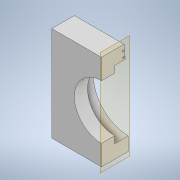
# Autodesk Inventor part: irrigation02
Saved by Autodesk Inventor 2021.1 (Build 251245000, 245)
## iProperties
Created: 2020-08-29
Part Number: irrigation02
Material: Generic
Document SubType Name: Modeling
Designer: robst
Density: 1 g/cm^3
Appearance: Default
Author: robst
Autodesk Inventor part; units mm, degrees
ref_plane "XZ Plane" through (0, 0, 0) normal (0, 1, 0) x (-1, 0, 0)
sketch "Sketch1" plane through (0, 0, 0) normal (1, 0, 0) x (0, 1, 0)
  line L0 (0, 0) -> (0, 12.7)
  line L1 (0, 0) -> (-101.6, 0) construction
  arc A0 (-101.6, 0) -> (0, 0) centre (-50.8, 556.4861) ccw
  line L2 (-50.8, -2.3139) -> (-50.8, 0) construction
  line L3 (0, 12.7) -> (101.6, 12.7) construction
  arc A1 (0, 12.7) -> (101.6, 12.7) centre (50.8, 569.1861) ccw
  line L4 (0, 12.7) -> (-53.34, 12.7)
  line L5 (-53.34, 12.7) -> (-53.34, -2.3081)
  dimension "d0" = 12.7
  dimension "d1" = 101.6
  dimension "d5" = 558.8
  dimension "d6" = 101.6
  dimension "d7" = 558.8
  dimension "d8" = 53.34
  constraints: 12 end point, 6 point on circle, 3 horizontal, 2 centre point, 1 midpoint, 1 perpendicular, 1 vertical
  measures "d0" distance of L0.start L0.end
  measures "d1" distance of L0.start L1.end
  measures "d5" radius of A0
  measures "d6" distance of L0.end L3.end
  measures "d7" radius of A1
  measures "d8" distance of L0.end L4.end
extrude "Extrusion1" add sketch "Sketch1" along normal mid plane 55.88
sketch "Sketch2" plane through (-27.94, -53.34, 12.7) normal (0, 0, 1) x (1, 0, 0)
  line L0 (27.94, 53.34) -> (27.94, 0) construction
  line L1 (0, 0) -> (55.88, 0) construction
  circle A0 centre (27.94, 26.67) radius 15.24
  line L2 (0, 53.34) -> (55.88, 53.34) projected
  dimension "d11" = 30.48
  dimension "d12" = 26.67
  constraints: 2 end point, 2 midpoint, 1 centre point
  measures "d11" diameter of A0
  measures "d12" distance from line of A0.centre L2
extrude "Extrusion2" cut sketch "Sketch2" against normal through all
ref_plane "Work Plane2" through (0, -50.8, -2.3139) normal (0, 0, 1) x (1, 0, 0)
sketch "Sketch3" plane through (0, -50.8, -2.3139) normal (0, 0, 1) x (1, 0, 0)
  spline S0 degree 2 poles (15.24, 24.13) (15.24, 50.5265) (-7.62, 37.3282) (-30.48, 24.13) (-7.62, 10.9318) (15.24, -2.2665) (15.24, 24.13) knots 0 0 0 0.333333 0.333333 0.666667 0.666667 1 1 1 weights 1 0.5 1 0.5 1 0.5 1 projected
  circle A0 centre (0, 24.13) radius 15.24 projected
  circle A1 centre (0, 24.13) radius 19.05
  point P0 (0, 50.8)
  dimension "d15" = 3.81
  constraints: 1 centre point, 1 coincident, 1 vertical alignment, 1 other
extrude "Extrusion3" cut sketch "Sketch3" along normal blind 7.62
sketch "Sketch4" plane through (0, -50.8, -2.3139) normal (0, 0, 1) x (1, 0, 0)
  line L0 (27.94, -2.54) -> (27.94, 50.8) construction
  line L1 (27.94, 46.355) -> (-26.8216, 46.355) construction
  line L2 (-27.94, 50.8) -> (27.94, 50.8) construction
  line L3 (18.0299, 44.45) -> (18.0299, 47.8092)
  line L4 (18.0299, 47.8092) -> (19.3081, 47.8092)
  line L5 (19.3081, 47.8092) -> (19.3081, 48.26)
  line L6 (19.3081, 48.26) -> (16.2453, 48.26)
  line L7 (16.2453, 48.26) -> (16.2453, 47.8092)
  line L8 (16.2453, 47.8092) -> (17.5236, 47.8092)
  line L9 (17.5236, 47.8092) -> (17.5236, 44.45)
  line L10 (17.5236, 44.45) -> (18.0299, 44.45)
  spline S0 degree 2 poles (13.1609, 47.8247) (12.9448, 47.5715) (12.7039, 46.8305) (12.7039, 46.355) knots 0 0 0 1 2 2 2
  spline S1 degree 2 poles (12.7039, 46.355) (12.7039, 45.8919) (12.9386, 45.1416) (13.1609, 44.8884) knots 0 0 0 1 2 2 2
  spline S2 degree 2 poles (13.1609, 44.8884) (13.3955, 44.6229) (14.0161, 44.3697) (14.3897, 44.3697) knots 0 0 0 1 2 2 2
  spline S3 degree 2 poles (14.3897, 44.3697) (14.7757, 44.3697) (15.3932, 44.6322) (15.6186, 44.8884) knots 0 0 0 1 2 2 2
  spline S4 degree 2 poles (15.6186, 44.8884) (15.8378, 45.1416) (16.0724, 45.8857) (16.0724, 46.355) knots 0 0 0 1 2 2 2
  spline S5 degree 2 poles (16.0724, 46.355) (16.0724, 46.8336) (15.8347, 47.5622) (15.6155, 47.8247) knots 0 0 0 1 2 2 2
  spline S6 degree 2 poles (15.6155, 47.8247) (15.3932, 48.0778) (14.7726, 48.3403) (14.3897, 48.3403) knots 0 0 0 1 2 2 2
  spline S7 degree 2 poles (14.3897, 48.3403) (14.0007, 48.3403) (13.377, 48.0686) (13.1609, 47.8247) knots 0 0 0 1 2 2 2
  spline S8 degree 2 poles (13.2319, 46.355) (13.2319, 46.7317) (13.3955, 47.3152) (13.5437, 47.5066) knots 0 0 0 1 2 2 2
  spline S9 degree 2 poles (13.5437, 47.5066) (13.695, 47.7042) (14.1211, 47.9018) (14.3866, 47.9018) knots 0 0 0 1 2 2 2
  spline S10 degree 2 poles (14.3866, 47.9018) (14.6614, 47.9018) (15.0752, 47.7104) (15.2326, 47.5066) knots 0 0 0 1 2 2 2
  spline S11 degree 2 poles (15.2326, 47.5066) (15.3839, 47.3121) (15.5445, 46.7255) (15.5445, 46.355) knots 0 0 0 1 2 2 2
  spline S12 degree 2 poles (15.5445, 46.355) (15.5445, 45.6047) (14.9146, 44.8082) (14.3866, 44.8082) knots 0 0 0 1 2 2 2
  spline S13 degree 2 poles (14.3866, 44.8082) (13.8587, 44.8082) (13.2319, 45.6047) (13.2319, 46.355) knots 0 0 0 1 2 2 2
  spline S14 degree 2 poles (9.7399, 47.1114) (9.7399, 46.8644) (9.9159, 46.4198) (10.0734, 46.2655) knots 0 0 0 1 2 2 2
  spline S15 degree 2 poles (10.0734, 46.2655) (10.271, 46.0709) (10.8051, 45.8703) (11.2127, 45.8703) knots 0 0 0 1 2 2 2
  line L11 (11.2127, 45.8703) -> (11.6418, 45.8703)
  line L12 (11.6418, 45.8703) -> (11.6418, 44.45)
  line L13 (11.6418, 44.45) -> (12.1482, 44.45)
  line L14 (12.1482, 44.45) -> (12.1482, 48.26)
  line L15 (12.1482, 48.26) -> (11.1911, 48.26)
  spline S16 degree 2 poles (11.1911, 48.26) (10.8514, 48.26) (10.3759, 48.1488) (10.1938, 48.0223) knots 0 0 0 1 2 2 2
  spline S17 degree 2 poles (10.1938, 48.0223) (9.9807, 47.8771) (9.7399, 47.4295) (9.7399, 47.1114) knots 0 0 0 1 2 2 2
  spline S18 degree 2 poles (10.2679, 47.096) (10.2679, 47.2936) (10.4037, 47.5838) (10.5427, 47.6765) knots 0 0 0 1 2 2 2
  spline S19 degree 2 poles (10.5427, 47.6765) (10.6631, 47.7567) (10.9842, 47.8216) (11.2219, 47.8216) knots 0 0 0 1 2 2 2
  line L16 (11.2219, 47.8216) -> (11.6418, 47.8216)
  line L17 (11.6418, 47.8216) -> (11.6418, 46.3025)
  line L18 (11.6418, 46.3025) -> (11.296, 46.3025)
  spline S20 degree 2 poles (11.296, 46.3025) (10.9873, 46.3025) (10.6075, 46.4013) (10.484, 46.531) knots 0 0 0 1 2 2 2
  spline S21 degree 2 poles (10.484, 46.531) (10.3698, 46.6452) (10.2679, 46.9138) (10.2679, 47.096) knots 0 0 0 1 2 2 2
  line L19 (7.7824, 48.4298) -> (9.2737, 43.6225)
  line L20 (9.2737, 43.6225) -> (9.706, 43.6225)
  line L21 (9.706, 43.6225) -> (8.2209, 48.4298)
  line L22 (8.2209, 48.4298) -> (7.7824, 48.4298)
  spline S22 degree 2 poles (4.6702, 45.6202) (4.6702, 45.3361) (4.8863, 44.9008) (5.0654, 44.7588) knots 0 0 0 1 2 2 2
  spline S23 degree 2 poles (5.0654, 44.7588) (5.2815, 44.592) (5.7725, 44.45) (6.1615, 44.45) knots 0 0 0 1 2 2 2
  line L23 (6.1615, 44.45) -> (7.2545, 44.45)
  line L24 (7.2545, 44.45) -> (7.2545, 48.26)
  line L25 (7.2545, 48.26) -> (6.2448, 48.26)
  spline S24 degree 2 poles (6.2448, 48.26) (5.8373, 48.26) (5.4297, 48.2075) (5.2445, 48.1056) knots 0 0 0 1 2 2 2
  spline S25 degree 2 poles (5.2445, 48.1056) (5.0376, 47.9976) (4.8493, 47.6425) (4.8493, 47.4017) knots 0 0 0 1 2 2 2
  spline S26 degree 2 poles (4.8493, 47.4017) (4.8493, 47.1331) (5.1333, 46.707) (5.3834, 46.5866) knots 0 0 0 1 2 2 2
  line L26 (5.3834, 46.5866) -> (5.3834, 46.568)
  spline S27 degree 2 poles (5.3834, 46.568) (5.0438, 46.4754) (4.6702, 45.9845) (4.6702, 45.6202) knots 0 0 0 1 2 2 2
  spline S28 degree 2 poles (5.1982, 45.5986) (5.1982, 45.8147) (5.3217, 46.0926) (5.5069, 46.1914) knots 0 0 0 1 2 2 2
  spline S29 degree 2 poles (5.5069, 46.1914) (5.6273, 46.2531) (5.9114, 46.2902) (6.1738, 46.2902) knots 0 0 0 1 2 2 2
  line L27 (6.1738, 46.2902) -> (6.7481, 46.2902)
  line L28 (6.7481, 46.2902) -> (6.7481, 44.8823)
  line L29 (6.7481, 44.8823) -> (6.3375, 44.8823)
  spline S30 degree 2 poles (6.3375, 44.8823) (6.004, 44.8823) (5.6212, 44.944) (5.473, 45.0428) knots 0 0 0 1 2 2 2
  spline S31 degree 2 poles (5.473, 45.0428) (5.3309, 45.1447) (5.1982, 45.3979) (5.1982, 45.5986) knots 0 0 0 1 2 2 2
  spline S32 degree 2 poles (5.3773, 47.3307) (5.3773, 47.4665) (5.4699, 47.6703) (5.5718, 47.7289) knots 0 0 0 1 2 2 2
  spline S33 degree 2 poles (5.5718, 47.7289) (5.6953, 47.7969) (5.9948, 47.8277) (6.2634, 47.8277) knots 0 0 0 1 2 2 2
  line L30 (6.2634, 47.8277) -> (6.7481, 47.8277)
  line L31 (6.7481, 47.8277) -> (6.7481, 46.7132)
  line L32 (6.7481, 46.7132) -> (6.1738, 46.7132)
  spline S34 degree 2 poles (6.1738, 46.7132) (5.9361, 46.7132) (5.7107, 46.7626) (5.5903, 46.8397) knots 0 0 0 1 2 2 2
  spline S35 degree 2 poles (5.5903, 46.8397) (5.473, 46.9138) (5.3773, 47.1516) (5.3773, 47.3307) knots 0 0 0 1 2 2 2
  line L33 (4.5776, 44.45) -> (3.2932, 48.26)
  line L34 (3.2932, 48.26) -> (2.6695, 48.26)
  line L35 (2.6695, 48.26) -> (1.3851, 44.45)
  line L36 (1.3851, 44.45) -> (1.9192, 44.45)
  line L37 (1.9192, 44.45) -> (2.265, 45.5152)
  line L38 (2.265, 45.5152) -> (3.7193, 45.5152)
  line L39 (3.7193, 45.5152) -> (4.0651, 44.45)
  line L40 (4.0651, 44.45) -> (4.5776, 44.45)
  line L41 (2.404, 45.9474) -> (2.9937, 47.7413)
  line L42 (2.9937, 47.7413) -> (3.5803, 45.9474)
  line L43 (3.5803, 45.9474) -> (2.404, 45.9474)
  spline S36 degree 2 poles (-0.5137, 44.3821) (-0.1432, 44.3821) (0.4835, 44.6322) (0.712, 44.8823) knots 0 0 0 1 2 2 2
  spline S37 degree 2 poles (0.712, 44.8823) (0.9405, 45.1293) (1.1906, 45.8703) (1.1906, 46.3519) knots 0 0 0 1 2 2 2
  spline S38 degree 2 poles (1.1906, 46.3519) (1.1906, 46.8305) (0.9467, 47.5406) (0.7151, 47.803) knots 0 0 0 1 2 2 2
  spline S39 degree 2 poles (0.7151, 47.803) (0.4866, 48.0593) (-0.1371, 48.3279) (-0.523, 48.3279) knots 0 0 0 1 2 2 2
  spline S40 degree 2 poles (-0.523, 48.3279) (-0.7144, 48.3279) (-1.051, 48.2724) (-1.193, 48.2291) knots 0 0 0 1 2 2 2
  spline S41 degree 2 poles (-1.193, 48.2291) (-1.3165, 48.189) (-1.5728, 48.0747) (-1.6993, 48.0068) knots 0 0 0 1 2 2 2
  line L44 (-1.6993, 48.0068) -> (-1.6993, 47.3955)
  line L45 (-1.6993, 47.3955) -> (-1.6592, 47.3955)
  spline S42 degree 2 poles (-1.6592, 47.3955) (-1.5913, 47.4572) (-1.3813, 47.6301) (-1.23, 47.7135) knots 0 0 0 1 2 2 2
  spline S43 degree 2 poles (-1.23, 47.7135) (-1.0849, 47.7938) (-0.7422, 47.8957) (-0.5199, 47.8957) knots 0 0 0 1 2 2 2
  spline S44 degree 2 poles (-0.5199, 47.8957) (-0.276, 47.8957) (0.1593, 47.695) (0.323, 47.5036) knots 0 0 0 1 2 2 2
  spline S45 degree 2 poles (0.323, 47.5036) (0.4835, 47.309) (0.6626, 46.7193) (0.6626, 46.3519) knots 0 0 0 1 2 2 2
  spline S46 degree 2 poles (0.6626, 46.3519) (0.6626, 45.9598) (0.4743, 45.3948) (0.3106, 45.2003) knots 0 0 0 1 2 2 2
  spline S47 degree 2 poles (0.3106, 45.2003) (0.1501, 45.0119) (-0.2791, 44.8205) (-0.5199, 44.8205) knots 0 0 0 1 2 2 2
  spline S48 degree 2 poles (-0.5199, 44.8205) (-0.7391, 44.8205) (-1.1127, 44.9286) (-1.2578, 45.0088) knots 0 0 0 1 2 2 2
  spline S49 degree 2 poles (-1.2578, 45.0088) (-1.3968, 45.0891) (-1.6036, 45.2558) (-1.6623, 45.3145) knots 0 0 0 1 2 2 2
  line L46 (-1.6623, 45.3145) -> (-1.6993, 45.3145)
  line L47 (-1.6993, 45.3145) -> (-1.6993, 44.7094)
  spline S50 degree 2 poles (-1.6993, 44.7094) (-1.5728, 44.6507) (-1.3505, 44.5426) (-1.193, 44.4932) knots 0 0 0 1 2 2 2
  spline S51 degree 2 poles (-1.193, 44.4932) (-1.0263, 44.4376) (-0.7422, 44.3821) (-0.5137, 44.3821) knots 0 0 0 1 2 2 2
  line L48 (-4.9505, 44.45) -> (-4.2929, 44.45)
  line L49 (-4.2929, 44.45) -> (-2.9004, 46.2222)
  line L50 (-2.9004, 46.2222) -> (-2.6781, 45.9721)
  line L51 (-2.6781, 45.9721) -> (-2.6781, 44.45)
  line L52 (-2.6781, 44.45) -> (-2.1717, 44.45)
  line L53 (-2.1717, 44.45) -> (-2.1717, 48.26)
  line L54 (-2.1717, 48.26) -> (-2.6781, 48.26)
  line L55 (-2.6781, 48.26) -> (-2.6781, 46.5094)
  line L56 (-2.6781, 46.5094) -> (-4.2404, 48.26)
  line L57 (-4.2404, 48.26) -> (-4.8579, 48.26)
  line L58 (-4.8579, 48.26) -> (-3.2802, 46.5588)
  line L59 (-3.2802, 46.5588) -> (-4.9505, 44.45)
  spline S52 degree 2 poles (-9.2977, 47.1114) (-9.2977, 46.8644) (-9.1217, 46.4198) (-8.9643, 46.2655) knots 0 0 0 1 2 2 2
  spline S53 degree 2 poles (-8.9643, 46.2655) (-8.7667, 46.0709) (-8.2325, 45.8703) (-7.825, 45.8703) knots 0 0 0 1 2 2 2
  line L60 (-7.825, 45.8703) -> (-7.3958, 45.8703)
  line L61 (-7.3958, 45.8703) -> (-7.3958, 44.45)
  line L62 (-7.3958, 44.45) -> (-6.8895, 44.45)
  line L63 (-6.8895, 44.45) -> (-6.8895, 48.26)
  line L64 (-6.8895, 48.26) -> (-7.8466, 48.26)
  spline S54 degree 2 poles (-7.8466, 48.26) (-8.1862, 48.26) (-8.6617, 48.1488) (-8.8439, 48.0223) knots 0 0 0 1 2 2 2
  spline S55 degree 2 poles (-8.8439, 48.0223) (-9.0569, 47.8771) (-9.2977, 47.4295) (-9.2977, 47.1114) knots 0 0 0 1 2 2 2
  spline S56 degree 2 poles (-8.7698, 47.096) (-8.7698, 47.2936) (-8.6339, 47.5838) (-8.495, 47.6765) knots 0 0 0 1 2 2 2
  spline S57 degree 2 poles (-8.495, 47.6765) (-8.3746, 47.7567) (-8.0535, 47.8216) (-7.8157, 47.8216) knots 0 0 0 1 2 2 2
  line L65 (-7.8157, 47.8216) -> (-7.3958, 47.8216)
  line L66 (-7.3958, 47.8216) -> (-7.3958, 46.3025)
  line L67 (-7.3958, 46.3025) -> (-7.7416, 46.3025)
  spline S58 degree 2 poles (-7.7416, 46.3025) (-8.0504, 46.3025) (-8.4301, 46.4013) (-8.5536, 46.531) knots 0 0 0 1 2 2 2
  spline S59 degree 2 poles (-8.5536, 46.531) (-8.6679, 46.6452) (-8.7698, 46.9138) (-8.7698, 47.096) knots 0 0 0 1 2 2 2
  line L68 (-12.5427, 48.26) -> (-11.2305, 44.45)
  line L69 (-11.2305, 44.45) -> (-10.684, 44.45)
  line L70 (-10.684, 44.45) -> (-9.3718, 48.26)
  line L71 (-9.3718, 48.26) -> (-9.9152, 48.26)
  line L72 (-9.9152, 48.26) -> (-10.9712, 45.0953)
  line L73 (-10.9712, 45.0953) -> (-12.0271, 48.26)
  line L74 (-12.0271, 48.26) -> (-12.5427, 48.26)
  spline S60 degree 2 poles (-15.2134, 46.355) (-15.2134, 45.3299) (-14.6175, 44.3697) (-13.9969, 44.3697) knots 0 0 0 1 2 2 2
  spline S61 degree 2 poles (-13.9969, 44.3697) (-13.3671, 44.3697) (-12.7774, 45.3485) (-12.7774, 46.3519) knots 0 0 0 1 2 2 2
  spline S62 degree 2 poles (-12.7774, 46.3519) (-12.7774, 47.3831) (-13.3733, 48.3372) (-13.9969, 48.3372) knots 0 0 0 1 2 2 2
  spline S63 degree 2 poles (-13.9969, 48.3372) (-14.6237, 48.3372) (-15.2134, 47.3492) (-15.2134, 46.355) knots 0 0 0 1 2 2 2
  spline S64 degree 2 poles (-14.5589, 45.1941) (-14.633, 45.3824) (-14.6947, 45.9629) (-14.6947, 46.355) knots 0 0 0 1 2 2 2
  spline S65 degree 2 poles (-14.6947, 46.355) (-14.6947, 46.7471) (-14.633, 47.3245) (-14.5558, 47.519) knots 0 0 0 1 2 2 2
  spline S66 degree 2 poles (-14.5558, 47.519) (-14.4786, 47.7135) (-14.21, 47.9142) (-13.9969, 47.9142) knots 0 0 0 1 2 2 2
  spline S67 degree 2 poles (-13.9969, 47.9142) (-13.7839, 47.9142) (-13.5091, 47.7135) (-13.4288, 47.5128) knots 0 0 0 1 2 2 2
  spline S68 degree 2 poles (-13.4288, 47.5128) (-13.3516, 47.3183) (-13.2961, 46.7255) (-13.2961, 46.3519) knots 0 0 0 1 2 2 2
  spline S69 degree 2 poles (-13.2961, 46.3519) (-13.2961, 45.9505) (-13.3455, 45.4133) (-13.4257, 45.2034) knots 0 0 0 1 2 2 2
  spline S70 degree 2 poles (-13.4257, 45.2034) (-13.4998, 45.0058) (-13.7746, 44.7927) (-13.9969, 44.7927) knots 0 0 0 1 2 2 2
  spline S71 degree 2 poles (-13.9969, 44.7927) (-14.2069, 44.7927) (-14.4817, 44.9934) (-14.5589, 45.1941) knots 0 0 0 1 2 2 2
  line L75 (-18.1527, 45.7591) -> (-17.6989, 45.7591)
  line L76 (-17.6989, 45.7591) -> (-17.6989, 44.45)
  line L77 (-17.6989, 44.45) -> (-17.208, 44.45)
  line L78 (-17.208, 44.45) -> (-17.208, 45.7591)
  line L79 (-17.208, 45.7591) -> (-15.5253, 45.7591)
  line L80 (-15.5253, 45.7591) -> (-15.5253, 46.2963)
  line L81 (-15.5253, 46.2963) -> (-17.2296, 48.26)
  line L82 (-17.2296, 48.26) -> (-17.6989, 48.26)
  line L83 (-17.6989, 48.26) -> (-17.6989, 46.1697)
  line L84 (-17.6989, 46.1697) -> (-18.1527, 46.1697)
  line L85 (-18.1527, 46.1697) -> (-18.1527, 45.7591)
  line L86 (-17.208, 46.1697) -> (-17.208, 47.6579)
  line L87 (-17.208, 47.6579) -> (-15.9266, 46.1697)
  line L88 (-15.9266, 46.1697) -> (-17.208, 46.1697)
  point P0 (0, 50.8)
  dimension "d18" = 4.445
  constraints: 2 end point, 2 horizontal, 1 point on line
  measures "d18" distance between parallel lines of L1 L2
emboss "Emboss1" sketch "Sketch4" operation cut depth 1.27 direction (0, 0, -1) wrap yes faces at (0.4387, -50.7848, -2.3139)
split "Split1" plane through (0, 0, 0) removes the side toward (1, 0, 0)
equation "\"d0\" = sidingDepth"
equation "\"d1\" = sidingHeight"
equation "\"d5\" = radiusOfCurvature"
equation "\"d6\" = sidingHeight"
equation "\"d7\" = radiusOfCurvature"
equation "\"d8\" = partHeight"
equation "\"d9\" = partWidth"
equation "\"d11\" = pipeDiameter"
equation "\"d12\" = pipeCenter"
equation "\"d15\" = clearanceRingForBackHole"
equation "\"d16\" = clearanceDepth"
equation "\"d18\" = textLine"
equation "\"d19\" = textDepth"
equation "\"sidingHeight\" = 101.6"
equation "\"sidingDepth\" = 12.7"
equation "\"radiusOfCurvature\" = 558.8"
equation "\"pipeDiameter\" = 30.48"
equation "\"partWidth\" = 55.88"
equation "\"partHeight\" = 53.34"
equation "\"pipeCenter\" = 26.67"
equation "\"clearanceRingForBackHole\" = 3.81"
equation "\"clearanceDepth\" = 7.62"
equation "\"textLine\" = 4.445"
equation "\"textDepth\" = 1.27"
body "Solid1"
